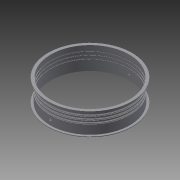
# Autodesk Inventor part: Rotation
Saved by Autodesk Inventor 2015 (Build 190159000, 159)
## iProperties
Created: 2015-06-16
Part Number: Rotation
Material: Generic
Document SubType Name: Modeling
Designer: david_000
Density: 1 g/cm^3
Appearance: Default
Author: david_000
Autodesk Inventor part; units mm, degrees
ref_plane "YZ Plane" through (0, 0, 0) normal (1, 0, 0) x (0, 1, 0)
ref_plane "XZ Plane" through (0, 0, 0) normal (0, 1, 0) x (-1, 0, 0)
ref_plane "XY Plane" through (0, 0, 0) normal (0, 0, 1) x (1, 0, 0)
sketch "Sketch1" plane through (0, 0, 0) normal (1, 0, 0) x (0, 1, 0)
  line L0 (25.4, 0) -> (25.4, -3.175)
  line L1 (0, -3.175) -> (0, 0)
  line L2 (0.635, 0) -> (0.635, -2.413)
  line L3 (24.765, -1.143) -> (24.765, 0)
  line L4 (0, 0) -> (0.635, 0)
  line L5 (24.765, 0) -> (25.4, 0)
  line L6 (18.415, -2.413) -> (18.415, -2.921)
  line L7 (18.415, -2.921) -> (20.955, -2.921)
  line L8 (20.955, -2.921) -> (20.955, -2.413)
  line L9 (10.795, -2.413) -> (10.795, -2.921)
  line L10 (10.795, -2.921) -> (13.335, -2.921)
  line L11 (13.335, -2.921) -> (13.335, -2.413)
  line L12 (14.5757, -2.413) -> (14.5757, -2.921)
  line L13 (14.5757, -2.921) -> (17.145, -2.921)
  line L14 (17.145, -2.921) -> (17.145, -2.413)
  line L15 (23.495, -2.413) -> (23.495, -1.143)
  line L16 (23.495, -1.143) -> (24.765, -1.143)
  line L17 (20.955, -2.413) -> (23.495, -2.413)
  line L18 (17.145, -2.413) -> (18.415, -2.413)
  line L19 (13.335, -2.413) -> (14.5757, -2.413)
  line L20 (20.32, -2.921) -> (19.05, -2.921)
  line L21 (19.05, -2.921) -> (19.05, -3.175)
  line L22 (19.05, -3.175) -> (20.32, -3.175)
  line L23 (20.32, -3.175) -> (20.32, -2.921)
  line L24 (15.2107, -2.921) -> (16.4807, -2.921)
  line L25 (16.4807, -2.921) -> (16.4807, -3.175)
  line L26 (16.4807, -3.175) -> (15.2107, -3.175)
  line L27 (15.2107, -3.175) -> (15.2107, -2.921)
  line L28 (11.43, -2.921) -> (12.7, -2.921)
  line L29 (12.7, -2.921) -> (12.7, -3.175)
  line L30 (12.7, -3.175) -> (11.43, -3.175)
  line L31 (11.43, -3.175) -> (11.43, -2.921)
  line L32 (0.635, -47.625) -> (20.32, -47.625)
  line L33 (25.4, -3.175) -> (7.62, -3.175)
  line L34 (5.08, -3.175) -> (0, -3.175)
  line L35 (0.635, -2.413) -> (5.08, -2.413)
  line L36 (7.62, -2.413) -> (10.795, -2.413)
  line L37 (7.62, -3.175) -> (5.08, -3.175)
  line L38 (5.08, -2.413) -> (7.62, -2.413)
  dimension "d3" = 2.413
  dimension "d21" = 1.27
  dimension "d22" = 0.254
  dimension "d23" = 1.27
  dimension "d24" = 0.254
  dimension "d25" = 1.27
  dimension "d26" = 0.254
  dimension "d27" = 0.635
  dimension "d28" = 0
  dimension "d56" = 0.635
  dimension "d57" = 0
  dimension "d59" = 0.635
  dimension "d60" = 0
  dimension "d78" = 0.762
  dimension "d106" = 25.4
  dimension "d107" = 24.765
  dimension "d108" = 23.495
  dimension "d109" = 20.955
  dimension "d110" = 18.415
  dimension "d111" = 17.145
  dimension "d112" = 14.5757
  dimension "d113" = 13.335
  dimension "d118" = 0.635
  dimension "d120" = 47.625
  dimension "d121" = 90
  dimension "d122" = 90
  dimension "d123" = 12.7
  dimension "d124" = 1.143
  dimension "d125" = 2.921
  dimension "d126" = 2.413
  dimension "d127" = 2.921
  dimension "d128" = 3.175
  dimension "d129" = 2.921
  dimension "d130" = 2.413
  dimension "d131" = 3.175
  dimension "d132" = 2.413
  dimension "d133" = 2.413
  dimension "d134" = 5.08
  dimension "d135" = 24.765
  dimension "d136" = 10.795
  dimension "d137" = 5.08
  constraints: 78 end point, 20 parallel, 5 horizontal, 4 collinear, 3 perpendicular
  measures "d3" distance of L2.end L2.start
  measures "d21" distance of L22.end L21.end
  measures "d22" distance of L21.end L20.end
  measures "d23" distance of L25.end L26.end
  measures "d24" distance of L24.end L25.end
  measures "d25" distance of L29.end L30.end
  measures "d26" distance of L28.end L29.end
  measures "d27" distance between parallel lines of L6 L21
  measures "d28" distance between parallel lines of L7 L20
  measures "d56" distance between parallel lines of L12 L27
  measures "d57" distance between parallel lines of L13 L24
  measures "d59" distance between parallel lines of L9 L31
  measures "d60" distance between parallel lines of L10 L28
  measures "d78" distance of L36.start L33.end
  measures "d106" distance between parallel lines of L1 L0
  measures "d107" distance between parallel lines of L1 L3
  measures "d108" distance between parallel lines of L1 L15
  measures "d109" distance between parallel lines of L1 L8
  measures "d110" distance between parallel lines of L1 L6
  measures "d111" distance between parallel lines of L1 L14
  measures "d112" distance between parallel lines of L1 L12
  measures "d113" distance between parallel lines of L1 L11
  measures "d118" distance between parallel lines of L1 L2
  measures "d120" distance from line of L3.end L32
  measures "d121" angle of L0 L17
  measures "d122" angle of L0 L19
  measures "d123" distance between parallel lines of L0 L29
  measures "d124" distance between parallel lines of L5 L16
  measures "d125" distance between parallel lines of L5 L20
  measures "d126" distance between parallel lines of L5 L18
  measures "d127" distance between parallel lines of L5 L13
  measures "d128" distance between parallel lines of L5 L33
  measures "d129" distance between parallel lines of L5 L10
  measures "d130" distance between parallel lines of L5 L35
  measures "d131" distance between parallel lines of L5 L34
  measures "d132" distance from line of L1.end L17
  measures "d133" distance from line of L1.end L19
  measures "d134" distance from line of L32.end L0
  measures "d135" distance from line of L32.start L0
  measures "d136" distance between parallel lines of L1 L9
  measures "d137" distance from line of L1 L34.start
revolve "Revolution1" add sketch "Sketch1" angle 360 about axis through (0, 0.635, -47.625) along (0, 1, 0) contours L0 L33 L23 L7 L8 L17 L15 L16 L3 L5 | L33 L25 L13 L14 L18 L6 L7 L21 | L33 L29 L10 L11 L19 L12 L13 L27 | L33 L37 L34 L1 L4 L2 L35 L38 L36 L9 L10 L31
sketch "Sketch2" plane through (0, 23.495, -47.625) normal (0, -1, 0) x (1, 0, 0)
  line L0 (0.0276, 45.212) -> (0.0276, 46.4905)
  line L1 (-2.3347, 45.1517) -> (-2.3984, 46.3675)
  line L2 (0.0352, 22.3605) -> (23.8944, 22.3605) construction
  line L3 (0.0276, 46.4905) -> (-2.3984, 46.3675)
  circle A0 centre (0, 0) radius 45.212 projected
  line L4 (0.0276, 45.212) -> (-2.3347, 45.1517)
  line L5 (-2.443, 45.0772) -> (-2.5813, 46.3483)
  line L6 (-4.785, 44.7618) -> (-4.9798, 45.9637)
  line L7 (-2.5813, 46.3483) -> (-4.9798, 45.9637)
  line L8 (-2.443, 45.0772) -> (-4.785, 44.7618)
  line L9 (-4.8846, 44.6761) -> (-5.1594, 45.9248)
  line L10 (-7.1787, 44.1094) -> (-7.5023, 45.2831)
  line L11 (-5.1594, 45.9248) -> (-7.5023, 45.2831)
  line L12 (-4.8846, 44.6761) -> (-7.1787, 44.1094)
  line L13 (-7.2685, 44.0134) -> (-7.6767, 45.225)
  line L14 (-9.4879, 43.2019) -> (-9.9365, 44.3337)
  line L15 (-7.6767, 45.225) -> (-9.9365, 44.3337)
  line L16 (-7.2685, 44.0134) -> (-9.4879, 43.2019)
  line L17 (-9.5668, 43.0968) -> (-10.1036, 44.2571)
  line L18 (-11.6854, 42.0501) -> (-12.2538, 43.1268)
  line L19 (-10.1036, 44.2571) -> (-12.2538, 43.1268)
  line L20 (-9.5668, 43.0968) -> (-11.6854, 42.0501)
  line L21 (-11.7524, 41.937) -> (-12.4116, 43.0326)
  line L22 (-13.7455, 40.6674) -> (-14.427, 41.6764)
  line L23 (-12.4116, 43.0326) -> (-14.427, 41.6764)
  line L24 (-11.7524, 41.937) -> (-13.7455, 40.6674)
  line L25 (-13.7999, 40.5478) -> (-14.5737, 41.5657)
  line L26 (-15.6441, 39.0702) -> (-16.4306, 39.9995)
  line L27 (-14.5737, 41.5657) -> (-16.4306, 39.9995)
  line L28 (-13.7999, 40.5478) -> (-15.6441, 39.0702)
  line L29 (-15.6852, 38.9453) -> (-16.5645, 39.8736)
  line L30 (-17.3588, 37.277) -> (-18.2412, 38.1159)
  line L31 (-16.5645, 39.8736) -> (-18.2412, 38.1159)
  line L32 (-15.6852, 38.9453) -> (-17.3588, 37.277)
  line L33 (-17.3862, 37.1484) -> (-18.3607, 37.9762)
  line L34 (-18.8696, 35.3089) -> (-19.8375, 36.0475)
  line L35 (-18.3607, 37.9762) -> (-19.8375, 36.0475)
  line L36 (-17.3862, 37.1484) -> (-18.8696, 35.3089)
  line L37 (-18.8829, 35.1782) -> (-19.9412, 35.8957)
  line L38 (-20.1587, 33.189) -> (-21.2008, 33.8186)
  line L39 (-19.9412, 35.8957) -> (-21.2008, 33.8186)
  line L40 (-18.8829, 35.1782) -> (-20.1587, 33.189)
  line L41 (-20.1579, 33.0576) -> (-21.2875, 33.6565)
  line L42 (-21.2111, 30.9422) -> (-22.3151, 31.4554)
  line L43 (-21.2875, 33.6565) -> (-22.3151, 31.4554)
  line L44 (-20.1579, 33.0576) -> (-21.2111, 30.9422)
  line L45 (-21.196, 30.8116) -> (-22.3838, 31.2849)
  line L46 (-22.0144, 28.5948) -> (-23.1675, 28.9856)
  line L47 (-22.3838, 31.2849) -> (-23.1675, 28.9856)
  line L48 (-21.196, 30.8116) -> (-22.0144, 28.5948)
  line L49 (-21.9853, 28.4666) -> (-23.2173, 28.8087)
  line L50 (-22.5592, 26.1742) -> (-23.7477, 26.4381)
  line L51 (-23.2173, 28.8087) -> (-23.7477, 26.4381)
  line L52 (-21.9853, 28.4666) -> (-22.5592, 26.1742)
  line L53 (-22.5164, 26.05) -> (-23.7781, 26.2568)
  line L54 (-22.8391, 23.709) -> (-24.0492, 23.8428)
  line L55 (-23.7781, 26.2568) -> (-24.0492, 23.8428)
  line L56 (-22.5164, 26.05) -> (-22.8391, 23.709)
  line L57 (-22.7831, 23.5901) -> (-24.0598, 23.6593)
  line L58 (-22.8508, 21.2279) -> (-24.0683, 21.2301)
  line L59 (-24.0598, 23.6593) -> (-24.0683, 21.2301)
  line L60 (-22.7831, 23.5901) -> (-22.8508, 21.2279)
  line L61 (-22.7823, 21.1158) -> (-24.0589, 21.0466)
  line L62 (-22.5941, 18.7602) -> (-23.8047, 18.6307)
  line L63 (-24.0589, 21.0466) -> (-23.8047, 18.6307)
  line L64 (-22.7823, 21.1158) -> (-22.5941, 18.7602)
  line L65 (-22.5139, 18.6561) -> (-23.7756, 18.4492)
  line L66 (-22.0722, 16.3346) -> (-23.2617, 16.075)
  line L67 (-23.7756, 18.4492) -> (-23.2617, 16.075)
  line L68 (-22.5139, 18.6561) -> (-22.0722, 16.3346)
  line L69 (-21.9812, 16.2398) -> (-23.2132, 15.8977)
  line L70 (-21.2911, 13.9797) -> (-22.4456, 13.593)
  line L71 (-23.2132, 15.8977) -> (-22.4456, 13.593)
  line L72 (-21.9812, 16.2398) -> (-21.2911, 13.9797)
  line L73 (-21.1904, 13.8953) -> (-22.3781, 13.422)
  line L74 (-20.26, 11.723) -> (-21.3659, 11.2138)
  line L75 (-22.3781, 13.422) -> (-21.3659, 11.2138)
  line L76 (-21.1904, 13.8953) -> (-20.26, 11.723)
  line L77 (-20.1507, 11.65) -> (-21.2803, 11.0511)
  line L78 (-18.9909, 9.5911) -> (-20.0352, 8.9653)
  line L79 (-21.2803, 11.0511) -> (-20.0352, 8.9653)
  line L80 (-20.1507, 11.65) -> (-18.9909, 9.5911)
  line L81 (-18.8744, 9.5303) -> (-19.9326, 8.8128)
  line L82 (-17.4987, 7.6089) -> (-18.4693, 6.8738)
  line L83 (-19.9326, 8.8128) -> (-18.4693, 6.8738)
  line L84 (-18.8744, 9.5303) -> (-17.4987, 7.6089)
  line L85 (-17.3763, 7.561) -> (-18.3508, 6.7333)
  line L86 (-15.801, 5.7996) -> (-16.6864, 4.9639)
  line L87 (-18.3508, 6.7333) -> (-16.6864, 4.9639)
  line L88 (-17.3763, 7.561) -> (-15.801, 5.7996)
  line L89 (-15.6741, 5.7653) -> (-16.5534, 4.837)
  line L90 (-13.9176, 4.1845) -> (-14.7075, 3.258)
  line L91 (-16.5534, 4.837) -> (-14.7075, 3.258)
  line L92 (-15.6741, 5.7653) -> (-13.9176, 4.1845)
  line L93 (-13.7878, 4.1641) -> (-14.5615, 3.1462)
  line L94 (-11.8706, 2.7824) -> (-12.5557, 1.776)
  line L95 (-14.5615, 3.1462) -> (-12.5557, 1.776)
  line L96 (-13.7878, 4.1641) -> (-11.8706, 2.7824)
  line L97 (-11.7394, 2.7762) -> (-12.3985, 1.6807)
  line L98 (-9.6841, 1.61) -> (-10.2563, 0.5353)
  line L99 (-12.3985, 1.6807) -> (-10.2563, 0.5353)
  line L100 (-11.7394, 2.7762) -> (-9.6841, 1.61)
  line L101 (-9.5529, 1.6179) -> (-10.0897, 0.4575)
  line L102 (-7.3836, 0.6808) -> (-7.8363, -0.4495)
  line L103 (-10.0897, 0.4575) -> (-7.8363, -0.4495)
  line L104 (-9.5529, 1.6179) -> (-7.3836, 0.6808)
  line L105 (-7.254, 0.7029) -> (-7.6623, -0.5088)
  line L106 (-4.9961, 0.0057) -> (-5.3239, -1.1668)
  line L107 (-7.6623, -0.5088) -> (-5.3239, -1.1668)
  line L108 (-7.254, 0.7029) -> (-4.9961, 0.0057)
  line L109 (-4.8697, 0.0417) -> (-5.1445, -1.2069)
  line L110 (-2.5496, -0.4072) -> (-2.7488, -1.6083)
  line L111 (-5.1445, -1.2069) -> (-2.7488, -1.6083)
  line L112 (-4.8697, 0.0417) -> (-2.5496, -0.4072)
  line L113 (-2.4278, -0.3578) -> (-2.5661, -1.6288)
  line L114 (-0.0728, -0.5532) -> (-0.1409, -1.7688)
  line L115 (-2.5661, -1.6288) -> (-0.1409, -1.7688)
  line L116 (-2.4278, -0.3578) -> (-0.0728, -0.5532)
  line L117 (0.0429, -0.4909) -> (0.0429, -1.7695)
  line L118 (2.4052, -0.4306) -> (2.4689, -1.6464)
  line L119 (0.0429, -1.7695) -> (2.4689, -1.6464)
  line L120 (0.0429, -0.4909) -> (2.4052, -0.4306)
  line L121 (2.5135, -0.3561) -> (2.6517, -1.6272)
  line L122 (4.8555, -0.0407) -> (5.0503, -1.2426)
  line L123 (2.6517, -1.6272) -> (5.0503, -1.2426)
  line L124 (2.5135, -0.3561) -> (4.8555, -0.0407)
  line L125 (4.9551, 0.045) -> (5.2299, -1.2037)
  line L126 (7.2492, 0.6117) -> (7.5728, -0.562)
  line L127 (5.2299, -1.2037) -> (7.5728, -0.562)
  line L128 (4.9551, 0.045) -> (7.2492, 0.6117)
  line L129 (7.339, 0.7077) -> (7.7472, -0.5039)
  line L130 (9.5584, 1.5192) -> (10.007, 0.3874)
  line L131 (7.7472, -0.5039) -> (10.007, 0.3874)
  line L132 (7.339, 0.7077) -> (9.5584, 1.5192)
  line L133 (9.6372, 1.6243) -> (10.1741, 0.464)
  line L134 (11.7559, 2.671) -> (12.3243, 1.5943)
  line L135 (10.1741, 0.464) -> (12.3243, 1.5943)
  line L136 (9.6372, 1.6243) -> (11.7559, 2.671)
  line L137 (11.8229, 2.7841) -> (12.4821, 1.6885)
  line L138 (13.816, 4.0537) -> (14.4974, 3.0447)
  line L139 (12.4821, 1.6885) -> (14.4974, 3.0447)
  line L140 (11.8229, 2.7841) -> (13.816, 4.0537)
  line L141 (13.8704, 4.1733) -> (14.6442, 3.1554)
  line L142 (15.7146, 5.6509) -> (16.5011, 4.7216)
  line L143 (14.6442, 3.1554) -> (16.5011, 4.7216)
  line L144 (13.8704, 4.1733) -> (15.7146, 5.6509)
  line L145 (15.7557, 5.7758) -> (16.635, 4.8475)
  line L146 (17.4293, 7.4441) -> (18.3117, 6.6052)
  line L147 (16.635, 4.8475) -> (18.3117, 6.6052)
  line L148 (15.7557, 5.7758) -> (17.4293, 7.4441)
  line L149 (17.4567, 7.5727) -> (18.4312, 6.7449)
  line L150 (18.9401, 9.4122) -> (19.908, 8.6736)
  line L151 (18.4312, 6.7449) -> (19.908, 8.6736)
  line L152 (17.4567, 7.5727) -> (18.9401, 9.4122)
  line L153 (18.9534, 9.5429) -> (20.0117, 8.8254)
  line L154 (20.2292, 11.5321) -> (21.2713, 10.9025)
  line L155 (20.0117, 8.8254) -> (21.2713, 10.9025)
  line L156 (18.9534, 9.5429) -> (20.2292, 11.5321)
  line L157 (20.2283, 11.6635) -> (21.358, 11.0646)
  line L158 (21.2816, 13.7789) -> (22.3856, 13.2657)
  line L159 (21.358, 11.0646) -> (22.3856, 13.2657)
  line L160 (20.2283, 11.6635) -> (21.2816, 13.7789)
  line L161 (21.2665, 13.9094) -> (22.4543, 13.4362)
  line L162 (22.0849, 16.1263) -> (23.238, 15.7355)
  line L163 (22.4543, 13.4362) -> (23.238, 15.7355)
  line L164 (21.2665, 13.9094) -> (22.0849, 16.1263)
  line L165 (22.0558, 16.2545) -> (23.2878, 15.9124)
  line L166 (22.6297, 18.5469) -> (23.8182, 18.283)
  line L167 (23.2878, 15.9124) -> (23.8182, 18.283)
  line L168 (22.0558, 16.2545) -> (22.6297, 18.5469)
  line L169 (22.5869, 18.6711) -> (23.8486, 18.4643)
  line L170 (22.9096, 21.0121) -> (24.1197, 20.8783)
  line L171 (23.8486, 18.4643) -> (24.1197, 20.8783)
  line L172 (22.5869, 18.6711) -> (22.9096, 21.0121)
  line L173 (22.8536, 21.131) -> (24.1303, 21.0618)
  line L174 (22.9213, 23.4932) -> (24.1388, 23.491)
  line L175 (24.1303, 21.0618) -> (24.1388, 23.491)
  line L176 (22.8536, 21.131) -> (22.9213, 23.4932)
  line L177 (22.8528, 23.6053) -> (24.1294, 23.6745)
  line L178 (22.6646, 25.9609) -> (23.8752, 26.0904)
  line L179 (24.1294, 23.6745) -> (23.8752, 26.0904)
  line L180 (22.8528, 23.6053) -> (22.6646, 25.9609)
  line L181 (22.5844, 26.065) -> (23.8461, 26.2719)
  line L182 (22.1427, 28.3865) -> (23.3322, 28.6461)
  line L183 (23.8461, 26.2719) -> (23.3322, 28.6461)
  line L184 (22.5844, 26.065) -> (22.1427, 28.3865)
  line L185 (22.0517, 28.4813) -> (23.2837, 28.8234)
  line L186 (21.3616, 30.7414) -> (22.5161, 31.1281)
  line L187 (23.2837, 28.8234) -> (22.5161, 31.1281)
  line L188 (22.0517, 28.4813) -> (21.3616, 30.7414)
  line L189 (21.2609, 30.8258) -> (22.4486, 31.2991)
  line L190 (20.3305, 32.9981) -> (21.4364, 33.5073)
  line L191 (22.4486, 31.2991) -> (21.4364, 33.5073)
  line L192 (21.2609, 30.8258) -> (20.3305, 32.9981)
  line L193 (20.2212, 33.0711) -> (21.3508, 33.67)
  line L194 (19.0614, 35.13) -> (20.1057, 35.7558)
  line L195 (21.3508, 33.67) -> (20.1057, 35.7558)
  line L196 (20.2212, 33.0711) -> (19.0614, 35.13)
  line L197 (18.9449, 35.1908) -> (20.0031, 35.9083)
  line L198 (17.5692, 37.1122) -> (18.5398, 37.8473)
  line L199 (20.0031, 35.9083) -> (18.5398, 37.8473)
  line L200 (18.9449, 35.1908) -> (17.5692, 37.1122)
  line L201 (17.4468, 37.1601) -> (18.4213, 37.9878)
  line L202 (15.8715, 38.9215) -> (16.7569, 39.7572)
  line L203 (18.4213, 37.9878) -> (16.7569, 39.7572)
  line L204 (17.4468, 37.1601) -> (15.8715, 38.9215)
  line L205 (15.7446, 38.9558) -> (16.6239, 39.8841)
  line L206 (13.9881, 40.5366) -> (14.778, 41.4631)
  line L207 (16.6239, 39.8841) -> (14.778, 41.4631)
  line L208 (15.7446, 38.9558) -> (13.9881, 40.5366)
  line L209 (13.8583, 40.557) -> (14.632, 41.5749)
  line L210 (11.9411, 41.9387) -> (12.6262, 42.9451)
  line L211 (14.632, 41.5749) -> (12.6262, 42.9451)
  line L212 (13.8583, 40.557) -> (11.9411, 41.9387)
  line L213 (11.8099, 41.9449) -> (12.469, 43.0404)
  line L214 (9.7546, 43.1111) -> (10.3268, 44.1858)
  line L215 (12.469, 43.0404) -> (10.3268, 44.1858)
  line L216 (11.8099, 41.9449) -> (9.7546, 43.1111)
  line L217 (9.6234, 43.1032) -> (10.1602, 44.2635)
  line L218 (7.4541, 44.0403) -> (7.9068, 45.1706)
  line L219 (10.1602, 44.2635) -> (7.9068, 45.1706)
  line L220 (9.6234, 43.1032) -> (7.4541, 44.0403)
  line L221 (7.3245, 44.0182) -> (7.7328, 45.2299)
  line L222 (5.0666, 44.7154) -> (5.3944, 45.8879)
  line L223 (7.7328, 45.2299) -> (5.3944, 45.8879)
  line L224 (7.3245, 44.0182) -> (5.0666, 44.7154)
  line L225 (4.9402, 44.6794) -> (5.215, 45.928)
  line L226 (2.6201, 45.1283) -> (2.8192, 46.3294)
  line L227 (5.215, 45.928) -> (2.8192, 46.3294)
  line L228 (4.9402, 44.6794) -> (2.6201, 45.1283)
  line L229 (2.4983, 45.0789) -> (2.6366, 46.3499)
  line L230 (0.1433, 45.2743) -> (0.2114, 46.4899)
  line L231 (2.6366, 46.3499) -> (0.2114, 46.4899)
  line L232 (2.4983, 45.0789) -> (0.1433, 45.2743)
  circle A1 centre (0, 0) radius 46.482 projected
  point P0 (0, 47.625)
  dimension "d62" = 24.13
  dimension "d63" = 24.13
  dimension "d64" = 93
  dimension "d67" = 360
  constraints: 466 end point, 2 point on circle, 1 horizontal, 1 vertical, 465 other
  measures "d62" distance of L2.start L0.end
  measures "d63" distance of L2.start L1.end
  measures "d64" angle of L2 L1
extrude "Extrusion1" cut sketch "Sketch2" against normal up to surface (1.27 mm away) contours A0 L1 L3 A1 L0 | A1 L3 L0 | L232 L230 A1 L231 L229 A0 | A0 L229 L232 | L230 L231 A1 | L5 L8 L6 A0 | A0 L6 L7 L5 | L226 L227 L225 A0 | A0 L225 L228 L226 | L9 L12 L10 A0 | A0 L10 L11 L9 | L222 L223 L221 A0 | A0 L221 L224 L222 | L13 L16 L14 A0 | A0 L14 L15 L13 | L218 L219 L217 A0 | A0 L217 L220 L218 | L17 L20 L18 L19 A0 | A0 L19 L17 | L214 L215 A0 | A0 L215 L213 L216 L214 | L24 L22 L23 L21 | L28 L26 L27 L25 | L32 L30 L31 L29 | L36 L34 L35 L33 | L40 L38 L39 L37 | L44 L42 L43 L41 | L48 L46 L47 L45 | L52 L50 L51 L49 | L56 L54 L55 L53 | L60 L58 L59 L57 | L64 L62 L63 L61 | L68 L66 L67 L65 | L72 L70 L71 L69 | L76 L74 L75 L73 | L80 L78 L79 L77 | L84 L82 L83 L81 | L88 L86 L87 L85 | L92 L90 L91 L89 | L96 L94 L95 L93 | L100 L98 L99 L97 | L104 L102 L103 L101 | L108 L106 L107 L105 | L112 L110 L111 L109 | L116 L114 L115 L113 | L120 L118 L119 L117 | L124 L122 L123 L121 | L128 L126 L127 L125 | L132 L130 L131 L129 | L136 L134 L135 L133 | L140 L138 L139 L137 | L144 L142 L143 L141 | L148 L146 L147 L145 | L152 L150 L151 L149 | L156 L154 L155 L153 | L160 L158 L159 L157 | L164 L162 L163 L161 | L168 L166 L167 L165 | L172 L170 L171 L169 | L176 L174 L175 L173 | L180 L178 L179 L177 | L184 L182 L183 L181 | L188 L186 L187 L185 | L192 L190 L191 L189 | L196 L194 L195 L193 | L200 L198 L199 L197 | L204 L202 L203 L201 | L208 L206 L207 L205 | L212 L210 L211 L209
ref_plane "Work Plane1" through (0, 7.62, -2.413) normal (0, 0, 1) x (1, 0, 0)
sketch "Sketch3" plane through (0, 7.62, -2.413) normal (0, 0, 1) x (1, 0, 0)
  line L0 (47.625, -7.62) -> (-47.625, -7.62) projected
  circle A0 centre (0, -1.27) radius 1.27
  point P0 (0, -7.62)
  dimension "d138" = 6.35
  dimension "d139" = 2.54
  constraints: 1 centre point, 1 coincident
  measures "d138" distance from line of L0 point (0, -1.27)
  measures "d139" diameter of A0
extrude "Extrusion2" cut sketch "Sketch3" against normal through all
body "Solid1"
